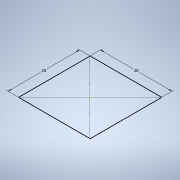
# Autodesk Inventor part: Stepper_Closing_2
Saved by Autodesk Inventor 2022.3 (Build 263350000, 350)
## iProperties
Created: 2023-05-23
Part Number: Stepper_Closing_2
Material: Generic
Document SubType Name: Modeling
Designer: Manuel Hueso Béjar
Density: 1 g/cm^3
Appearance: Default
Author: Manuel Hueso Béjar
Autodesk Inventor part; units mm, degrees
ref_plane "YZ Plane" through (0, 0, 0) normal (1, 0, 0) x (0, 1, 0)
ref_plane "XZ Plane" through (0, 0, 0) normal (0, 1, 0) x (-1, 0, 0)
ref_plane "XY Plane" through (0, 0, 0) normal (0, 0, 1) x (1, 0, 0)
sketch "Sketch1" plane through (0, 0, 0) normal (0, 1, 0) x (-1, 0, 0)
  line L0 (-22, 21.5) -> (22, 21.5)
  line L1 (22, 21.5) -> (22, -21.5)
  line L2 (22, -21.5) -> (-22, -21.5)
  line L3 (-22, -21.5) -> (-22, 21.5)
  line L4 (-22, 21.5) -> (22, -21.5) construction
  line L5 (22, 21.5) -> (-22, -21.5) construction
  line L6 (-22, 21.5) -> (-18, 21.5)
  line L7 (-18, 21.5) -> (-18, 12.5)
  line L8 (-18, 12.5) -> (-22, 12.5)
  line L9 (-22, 12.5) -> (-22, 21.5)
  line L10 (-22, -21.5) -> (-18, -21.5)
  line L11 (-18, -21.5) -> (-18, -12.5)
  line L12 (-18, -12.5) -> (-22, -12.5)
  line L13 (-22, -12.5) -> (-22, -21.5)
  point P0 (0, 0)
  point P1 (-22, 12.5)
  dimension "d0" = 44
  dimension "d1" = 43
  dimension "d7" = 4
  dimension "d8" = 9
  dimension "d9" = 4
  dimension "d10" = 9
  constraints: 28 end point, 6 parallel, 3 horizontal, 3 perpendicular, 2 midpoint
  measures "d0" distance of L1.end L2.end
  measures "d1" distance of L0.end L1.end
  measures "d7" distance of L7.end L8.end
  measures "d8" distance of L6.end L7.end
  measures "d9" distance of L12.end L11.end
  measures "d10" distance of L11.end L10.end
extrude "Extrusion1" add sketch "Sketch1" along normal blind 2 contours L0 L1 L2 L11 L12 L3 L8 L7
sketch "Sketch3" plane through (0, 2, 0) normal (0, 1, 0) x (1, 0, 0)
  line L0 (18, -12.5) -> (22, -12.5) projected
  line L1 (22, -12.5) -> (22, 12.5) projected
  line L2 (18, -12.5) -> (22, -12.5)
  line L3 (22, -12.5) -> (22, 12.5)
  line L4 (22, 12.5) -> (18, 12.5)
  line L5 (18, 12.5) -> (18, -12.5)
  point P0 (0, 0)
  constraints: 8 end point, 2 parallel, 1 horizontal, 1 perpendicular
extrude "Extrusion3" add sketch "Sketch3" against normal blind 30
sketch "Sketch4" plane through (22, 2, 12.5) normal (1, 0, 0) x (0, 0, -1)
  line L0 (0, -30) -> (25, -30) projected
  circle A0 centre (12.5, -30) radius 11.5
  point P0 (12.5, -2)
  dimension "d13" = 23
  constraints: 1 centre point, 1 midpoint
  measures "d13" diameter of A0
extrude "Extrusion4" cut sketch "Sketch4" against normal blind 4
sketch "Sketch5" plane through (0, 2, 0) normal (0, 1, 0) x (1, 0, 0)
  line L0 (-22, 21.5) -> (-22, -21.5) projected
  line L1 (-22, 0) -> (-14, 0)
  line L2 (-22, 0) -> (-14, 0) construction
  circle A0 centre (-14, 0) radius 6
  point P0 (0, 0)
  dimension "d16" = 8
  dimension "d17" = 0
  dimension "d18" = 12
  constraints: 4 end point, 1 centre point, 1 coincident, 1 collinear, 1 horizontal, 1 midpoint, 1 perpendicular
  measures "d16" distance of L1.start L1.end
  measures "d17" distance between parallel lines of L1 L2
  measures "d18" diameter of A0
extrude "Extrusion5" cut sketch "Sketch5" against normal through all
body "Solid1"
